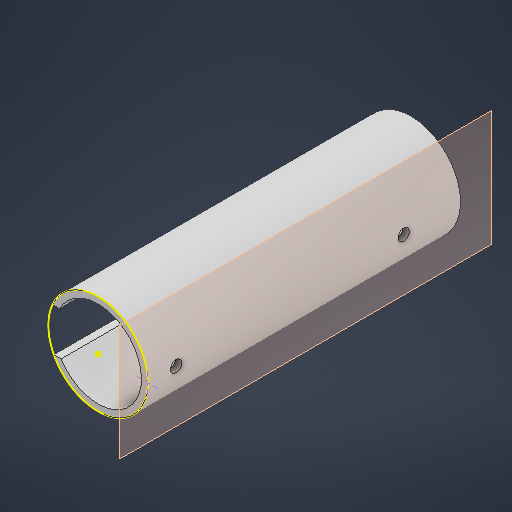
# Autodesk Inventor part: Solenoid Yoke
Saved by Autodesk Inventor 2026.3 (Build 303398000, 398)
## iProperties
Created: 2026-07-22
Part Number: Solenoid Yoke
Material: Generic
Document SubType Name: Sheet Metal
Designer: matot
Density: 1 g/cm^3
Sheet Metal Rule: Default_mm
Appearance: Default
Author: matot
Autodesk Inventor part; units mm, degrees
ref_plane "YZ Plane" through (0, 0, 0) normal (1, 0, 0) x (0, 1, 0)
ref_plane "XZ Plane" through (0, 0, 0) normal (0, 1, 0) x (-1, 0, 0)
ref_plane "XY Plane" through (0, 0, 0) normal (0, 0, 1) x (1, 0, 0)
sketch "Sketch1" plane through (0, 0, 0) normal (0, 0, 1) x (1, 0, 0)
  circle A0 centre (0, 0) radius 15.25
  circle A1 centre (0, 0) radius 17.5
  line L0 (-17.4453, -1.3829) -> (-17.4453, 0)
  line L1 (-17.9063, 7.789) -> (-15.9453, 7.789)
  line L2 (-15.9453, 7.789) -> (-15.9453, -7.211)
  line L3 (-15.9453, -7.211) -> (-17.9063, -7.211)
  line L4 (-17.9063, -7.211) -> (-17.9063, 7.789)
  line L5 (-17.9063, 7.789) -> (-15.9453, 7.789)
  line L6 (-15.9453, 7.789) -> (-15.9453, -7.211)
  line L7 (-15.9453, -7.211) -> (-17.9063, -7.211)
  line L8 (-17.9063, -7.211) -> (-17.9063, 7.789)
  point P0 (-15.9453, 0.289)
  dimension "d0" = 30.5
  dimension "d1" = 35
  dimension "d20" = 1.5
  constraints: 18 end point, 4 parallel, 2 centre point, 2 coincident, 2 horizontal, 2 perpendicular, 2 point on circle, 1 midpoint, 1 vertical
  measures "d0" diameter of A0
  measures "d1" diameter of A1
  measures "d20" horizontal distance of point (-15.945, 0.289) L0.end
extrude "Extrusion1" add sketch "Sketch1" along normal blind 110 contours A1 L2 | L2 A1
sketch "Sketch4" plane through (0, 0, 110) normal (0, 0, 1) x (1, 0, 0)
  circle A0 centre (0, 0) radius 17.5 projected
  point P0 (17.5, 0)
  constraints: 1 horizontal alignment, 1 other
sketch "Sketch6" plane through (0, 0, 110) normal (0, 0, 1) x (1, 0, 0)
  line L0 (-22.5, 7) -> (-12.5, 7)
  line L1 (-12.5, 7) -> (-12.5, -8)
  line L2 (-12.5, -8) -> (-22.5, -8)
  line L3 (-22.5, -8) -> (-22.5, 7)
  circle A0 centre (0, 0) radius 17.5 projected
  dimension "d21" = 5
  dimension "d24" = 10
  constraints: 8 end point, 2 parallel, 1 horizontal, 1 perpendicular
  measures "d21" distance edge to line of A0 L1
  measures "d24" distance between parallel lines of L3 L1
extrude "Extrusion4" cut sketch "Sketch6" against normal through all contours L0 A0 L2 L3 | L0 L1 L2 A0 picked at (-14.1637, -0.5178)
ref_plane "Work Plane2" through (17.5, 0, 110) normal (1, 0, 0) x (0, 1, 0)
sketch "Sketch7" plane through (17.5, 0, 110) normal (1, 0, 0) x (0, 1, 0)
  circle A0 centre (0, -10) radius 2
  circle A1 centre (0, -90) radius 2
  line L0 (17.5, 0) -> (-17.5, 0) projected
  point P0 (0, -110)
  point P1 (-8, 0)
  point P2 (7, 0)
  point P3 (0, 0)
  dimension "d25" = 10
  dimension "d26" = 80
  dimension "d27" = 4
  dimension "d28" = 4
  constraints: 2 centre point, 2 coincident, 1 midpoint
  measures "d25" distance of point (0, 0) A0.centre
  measures "d26" distance of A1.centre A0.centre
  measures "d27" diameter of A0
  measures "d28" diameter of A1
extrude "Extrusion5" cut sketch "Sketch7" against normal blind 10
equation "\"BendRadius\" = Thickness"
equation "\"BendReliefWidth\" = Thickness"
equation "\"BendReliefDepth\" = 0.5 * Thickness"
equation "\"CornerReliefSize\" = 4 * Thickness"
equation "\"MinimumRemnant\" = 2 * Thickness"
equation "\"TransitionRadius\" = BendRadius"
equation "\"JacobiRadiusSize\" = BendRadius"
equation "\"GapSize\" = Thickness"
equation "\"Thickness\" = 0.5"
body "Solid1"
